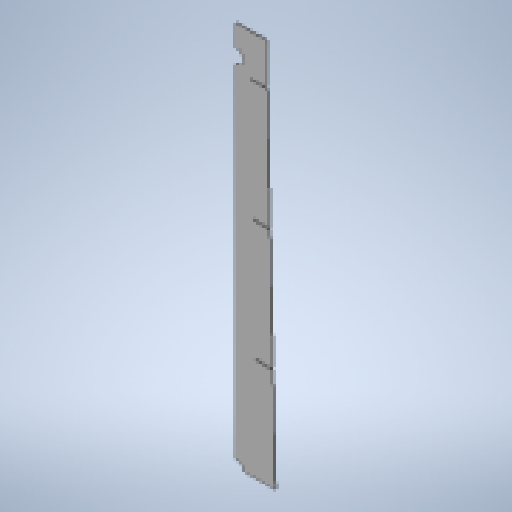
# Autodesk Inventor part: GBK 3212 central second rib
Saved by Autodesk Inventor 2026 (Build 300175000, 175)
## iProperties
Created: 2026-04-17
Part Number: GBK 3212 central second rib
Material: Steel
Document SubType Name: Sheet Metal
Designer: pokla
Mass: 7201.32 g
Surface Area: 4740.76 cm^2
Volume: 917.366 cm^3
Density: 7.85 g/cm^3
Flat Pattern Width: 16.2667 cm
Flat Pattern Length: 159.962 cm
Flat Pattern Area: 2602.06 cm^2
Sheet Metal Rule: По умолчанию
Sheet Metal Width: 162,667 мм
Sheet Metal Length: 1599,625 мм
Sheet Metal Area: 260205,598 мм^2
Appearance: Default
Author: admin
Autodesk Inventor part; units mm, degrees
ref_plane "YZ Plane" through (0, 0, 0) normal (1, 0, 0) x (0, 1, 0)
ref_plane "XZ Plane" through (0, 0, 0) normal (0, 1, 0) x (-1, 0, 0)
ref_plane "XY Plane" through (0, 0, 0) normal (0, 0, 1) x (1, 0, 0)
sketch "Sketch1" plane through (0, 0, 0) normal (0, 0, 1) x (1, 0, 0)
  line L0 (0, 0) -> (0, 4438.8737)
  line L1 (0, 4438.8737) -> (96, 4438.8737)
  line L2 (96, 4438.8737) -> (196, 0)
  line L3 (196, 0) -> (0, 0)
  circle A0 centre (0, 0) radius 30
  line L4 (0, 1479.6246) -> (162.6667, 1479.6246)
  line L5 (0, 2959.2492) -> (129.3333, 2959.2492)
  circle A1 centre (0, 1479.6246) radius 30
  circle A2 centre (0, 2959.2492) radius 30
  line L6 (186.8761, 405) -> (116.8761, 405)
  line L7 (116.8761, 405) -> (116.8761, 410)
  line L8 (116.8761, 410) -> (186.8761, 410)
  line L9 (186.8761, 410) -> (186.8761, 405)
  line L10 (105.6148, 909.8732) -> (175.6148, 909.8732)
  line L11 (175.6148, 904.8732) -> (105.6148, 904.8732)
  line L12 (105.6148, 904.8732) -> (105.6148, 909.8732)
  line L13 (175.6148, 909.8732) -> (175.6148, 904.8732)
  line L14 (94.3535, 1409.7463) -> (164.3535, 1409.7463)
  line L15 (164.3535, 1404.7463) -> (94.3535, 1404.7463)
  line L16 (94.3535, 1404.7463) -> (94.3535, 1409.7463)
  line L17 (164.3535, 1409.7463) -> (164.3535, 1404.7463)
  line L18 (83.0923, 1909.6195) -> (153.0923, 1909.6195)
  line L19 (153.0923, 1904.6195) -> (83.0923, 1904.6195)
  line L20 (83.0923, 1904.6195) -> (83.0923, 1909.6195)
  line L21 (153.0923, 1909.6195) -> (153.0923, 1904.6195)
  line L22 (71.831, 2409.4927) -> (141.831, 2409.4927)
  line L23 (141.831, 2404.4927) -> (71.831, 2404.4927)
  line L24 (71.831, 2404.4927) -> (71.831, 2409.4927)
  line L25 (141.831, 2409.4927) -> (141.831, 2404.4927)
  line L26 (60.5698, 2909.3658) -> (130.5698, 2909.3658)
  line L27 (130.5698, 2904.3658) -> (60.5698, 2904.3658)
  line L28 (60.5698, 2904.3658) -> (60.5698, 2909.3658)
  line L29 (130.5698, 2909.3658) -> (130.5698, 2904.3658)
  line L30 (49.3085, 3409.239) -> (119.3085, 3409.239)
  line L31 (119.3085, 3404.239) -> (49.3085, 3404.239)
  line L32 (49.3085, 3404.239) -> (49.3085, 3409.239)
  line L33 (119.3085, 3409.239) -> (119.3085, 3404.239)
  line L34 (38.0472, 3909.1122) -> (108.0472, 3909.1122)
  line L35 (108.0472, 3904.1122) -> (38.0472, 3904.1122)
  line L36 (38.0472, 3904.1122) -> (38.0472, 3909.1122)
  line L37 (108.0472, 3909.1122) -> (108.0472, 3904.1122)
  line L38 (0, 1629.6246) -> (159.2874, 1629.6246)
  line L39 (0, 3079.2492) -> (126.6299, 3079.2492)
  point P0 (30, 2959.2492)
  point P1 (0, 2929.2492)
  point P2 (0, 1509.6246)
  point P3 (0, 1449.6246)
  point P4 (0, 30)
  point P5 (30, 0)
  point P6 (186.7634, 410)
  point P7 (175.5022, 909.8732)
  point P8 (164.2409, 1409.7463)
  point P9 (30, 1479.6246)
  point P10 (153.0923, 1904.6195)
  point P11 (152.9796, 1909.6195)
  point P12 (141.831, 2404.4927)
  point P13 (141.7184, 2409.4927)
  point P14 (130.5698, 2904.3658)
  point P15 (130.4571, 2909.3658)
  point P16 (0, 2989.2492)
  dimension "d65" = 96
  dimension "d67" = 196
  dimension "d68" = 60
  dimension "d69" = 1480
  dimension "d70" = 1480
  dimension "d71" = 1480
  dimension "d72" = 5
  dimension "d73" = 70
  dimension "d74" = 410
  dimension "d77" = 500
  dimension "d82" = 120
  dimension "d83" = 150
  measures "d65" distance of L0.end L1.end
  measures "d67" distance of L2.end L0.start
  measures "d68" diameter of A0
  measures "d69" distance of L4.end L2.end
  measures "d70" distance of L4.end L5.end
  measures "d71" distance of L1.end L5.end
  measures "d72" distance of L6.end L7.end
  measures "d73" distance of L6.start L6.end
  measures "d74" distance between parallel lines of L3 L8
  measures "d77" distance of L7.end L10.start
  measures "d82" distance between parallel lines of L5 L39
  measures "d83" distance between parallel lines of L38 L4
extrude "Plate3" add sketch "Sketch1" along normal blind 4 contours L39 L2 L5 A2 L0 | L5 L2 L26 L28 L27 L22 L24 L23 L18 L20 L19 L38 L0 A2 | L38 L2 L4 A1 L0
chamfer "Corner Chamfer2" distance 3 angle 45 6 edges at (153.0923, 1904.6195, 2) (152.9796, 1909.6195, 2) (141.831, 2404.4927, 2) (141.7184, 2409.4927, 2) (130.5698, 2904.3658, 2) (130.4571, 2909.3658, 2)
equation "\"BendRadius\" = Thickness"
equation "\"BendReliefWidth\" = Thickness"
equation "\"BendReliefDepth\" = 0.5 * Thickness"
equation "\"CornerReliefSize\" = 4 * Thickness"
equation "\"MinimumRemnant\" = 2 * Thickness"
equation "\"TransitionRadius\" = BendRadius"
equation "\"JacobiRadiusSize\" = BendRadius"
equation "\"GapSize\" = Thickness"
equation "\"Thickness\" = 4"
body "Solid2"
